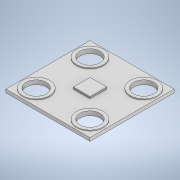
# Autodesk Inventor part: SiPM
Saved by Autodesk Inventor 2020 (Build 240168000, 168)
## iProperties
Created: 2021-06-25
Part Number: SiPM
Material: Generic
Document SubType Name: Modeling
Designer: alejandrosalazar
Density: 1 g/cm^3
Appearance: Default
Author: alejandrosalazar
Autodesk Inventor part; units mm, degrees
ref_plane "YZ Plane" through (0, 0, 0) normal (1, 0, 0) x (0, 1, 0)
ref_plane "XZ Plane" through (0, 0, 0) normal (0, 1, 0) x (-1, 0, 0)
ref_plane "XY Plane" through (0, 0, 0) normal (0, 0, 1) x (1, 0, 0)
sketch "Sketch1" plane through (0, 0, 0) normal (0, 1, 0) x (-1, 0, 0)
  line L0 (0, 0) -> (-25, 0)
  line L1 (-25, 0) -> (-25, 25)
  line L2 (-25, 25) -> (0, 25)
  line L3 (0, 25) -> (0, 0)
  circle A0 centre (-4.5, 4.5) radius 3
  circle A1 centre (-4.5, 20.5) radius 3
  circle A2 centre (-20.5, 20.5) radius 3
  circle A3 centre (-20.5, 4.5) radius 3
  dimension "d0" = 25
  dimension "d1" = 25
  dimension "d8" = 6
  dimension "d9" = 6
  dimension "d10" = 6
  dimension "d11" = 6
  constraints: 8 end point, 4 centre point, 2 parallel, 1 horizontal, 1 perpendicular
  measures "d0" distance of L1.end L2.end
  measures "d1" distance of L0.end L1.end
  measures "d8" diameter of A0
  measures "d9" diameter of A1
  measures "d10" diameter of A2
  measures "d11" diameter of A3
extrude "Extrusion1" add sketch "Sketch1" along normal blind 1 contours L0 L1 L2 L3 | A0 | A1 | A2 | A3
sketch "Sketch2" plane through (0, 1, 0) normal (0, 1, 0) x (1, 0, 0)
  line L0 (10, -12.5) -> (10, -15)
  line L1 (10, -15) -> (12.5, -15)
  line L2 (10, -12.5) -> (10, -10)
  line L3 (10, -10) -> (12.5, -10)
  line L4 (15, -12.5) -> (15, -15)
  line L5 (15, -15) -> (12.5, -15)
  line L6 (15, -12.5) -> (15, -10)
  line L7 (15, -10) -> (12.5, -10)
  point P0 (0, 0)
  dimension "d18" = 2.5
  dimension "d19" = 2.5
  dimension "d20" = 2.5
  dimension "d21" = 2.5
  dimension "d22" = 2.5
  dimension "d23" = 2.5
  constraints: 16 end point, 2 point on line
  measures "d18" distance of L1.end L0.end
  measures "d19" distance of L0.end L0.start
  measures "d20" distance of L2.end L3.end
  measures "d21" distance of L2.start L2.end
  measures "d22" distance of L4.end L5.end
  measures "d23" distance of L4.start L4.end
extrude "Extrusion2" add sketch "Sketch2" along normal blind 0.5
sketch "Sketch6" plane through (0, 1, 0) normal (0, 1, 0) x (1, 0, 0)
  circle A0 centre (4.5, -4.5) radius 4
  circle A1 centre (20.5, -4.5) radius 4
  circle A2 centre (4.5, -20.5) radius 4
  circle A3 centre (20.5, -20.5) radius 4
  point P0 (0, 0)
  dimension "d43" = 8
  dimension "d44" = 8
  dimension "d45" = 8
  dimension "d46" = 8
  constraints: 4 centre point
  measures "d43" diameter of A0
  measures "d44" diameter of A1
  measures "d45" diameter of A2
  measures "d46" diameter of A3
extrude "Extrusion4" add sketch "Sketch6" along normal blind 0.25
sketch "Sketch7" plane through (4.5, 1.25, 20.5) normal (0, 1, 0) x (1, 0, 0)
  circle A0 centre (0, 0) radius 3
  point P0 (-4.5, 20.5)
  dimension "d49" = 6
  constraints: 1 centre point
  measures "d49" diameter of A0
hole "Hole2" at (4.5, 1.25, 20.5) direction (0, -1, 0) diameter 6 depth 1.25
sketch "Sketch8" plane through (4.5, 1.25, 4.5) normal (0, 1, 0) x (1, 0, 0)
  circle A0 centre (0, 0) radius 3
  point P0 (-4.5, 4.5)
  dimension "d57" = 6
  constraints: 1 centre point
  measures "d57" diameter of A0
hole "Hole3" at (4.5, 1.25, 4.5) direction (0, -1, 0) diameter 6 depth 1.25
sketch "Sketch9" plane through (20.5, 1.25, 20.5) normal (0, 1, 0) x (1, 0, 0)
  circle A0 centre (0, 0) radius 3
  point P0 (-20.5, 20.5)
  dimension "d65" = 6
  constraints: 1 centre point
  measures "d65" diameter of A0
hole "Hole4" at (20.5, 1.25, 20.5) direction (0, -1, 0) diameter 6 depth 1.25
sketch "Sketch10" plane through (20.5, 1.25, 4.5) normal (0, 1, 0) x (1, 0, 0)
  circle A0 centre (0, 0) radius 3
  point P0 (-20.5, 4.5)
  dimension "d73" = 6
  constraints: 1 centre point
  measures "d73" diameter of A0
hole "Hole5" at (20.5, 1.25, 4.5) direction (0, -1, 0) diameter 6 depth 1.25
body "Solid1"
